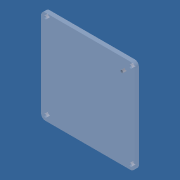
# Autodesk Inventor part: J007954
Saved by Autodesk Inventor 2018.2 (Build 222227000, 227)
## iProperties
Created: 2018-01-11
Material: ACRYLIC, CLEAR
Vendor: HHMI: JRC - ID&F
Document SubType Name: Modeling
Designer: negrashovi
Density: 0.66 g/cm^3
Appearance: Polycarbonate (Clear)
Project: P-159707
Description: WINDOW
Part Number: J007954
RuleStatus: InUse
AfterDocSave0: file://Part Number Cleaner
LAB/DEPT: RUBIN (LAB)
REQUESTING SCIENTIST: ASO, YOSHI
SURFACE ROUGHNESS: N/A
DESIGN DEPARTMENT: HHMI: JRC - ID&F
SPECIAL FINISH: NONE
ALTERED ITEM PART NUMBER: N/A
ALTERED ITEM VENDOR: N/A
ALTERED ITEM DESCRIPTION: N/A
Author: negrashovi
Revision Number: -
Autodesk Inventor part; units mm, degrees
ref_plane "YZ Plane" through (0, 0, 0) normal (1, 0, 0) x (0, 1, 0)
ref_plane "XZ Plane" through (0, 0, 0) normal (0, 1, 0) x (-1, 0, 0)
ref_plane "XY Plane" through (0, 0, 0) normal (0, 0, 1) x (1, 0, 0)
sketch "Sketch1" plane through (0, 0, 0) normal (0, 0, 1) x (1, 0, 0)
  line L0 (-63.5, -69.85) -> (63.5, -69.85)
  line L1 (69.85, -63.5) -> (69.85, 63.5)
  line L2 (63.5, 69.85) -> (-63.5, 69.85)
  line L3 (-69.85, 63.5) -> (-69.85, -63.5)
  arc A0 (-63.5, 69.85) -> (-69.85, 63.5) centre (-63.5, 63.5) ccw
  arc A1 (69.85, 63.5) -> (63.5, 69.85) centre (63.5, 63.5) ccw
  arc A2 (63.5, -69.85) -> (69.85, -63.5) centre (63.5, -63.5) ccw
  arc A3 (-69.85, -63.5) -> (-63.5, -69.85) centre (-63.5, -63.5) ccw
  point P0 (0, 0)
  point P1 (69.85, 0)
  point P2 (0, 69.85)
  point P3 (50.8, 50.8)
  dimension "d0" = 139.7
  dimension "d1" = 139.7
  dimension "d2" = 6.35
  dimension "d3" = 19.05
  dimension "d4" = 19.05
  constraints: 8 end point, 8 point on circle, 8 tangent, 4 centre point, 4 coincident, 3 equal radius, 2 midpoint, 2 parallel, 1 horizontal, 1 horizontal alignment, 1 perpendicular, 1 vertical alignment
  measures "d0" distance between parallel lines of L1 L3
  measures "d1" distance between parallel lines of L0 L2
  measures "d2" radius of A0
  measures "d3" distance from line of point (50.8, 50.8) L1
  measures "d4" distance from line of point (50.8, 50.8) L2
extrude "Extrusion1" add sketch "Sketch1" against normal blind 6.35
hole "Hole1" at (-63.5, 63.5, 0) at (63.5, 63.5, 0) at (63.5, -63.5, 0) at (-63.5, -63.5, 0) direction (0, 0, -1) diameter 4.4958 end through all clearance for "Flat Head Machine Screw (82)" size "#8" standard "Ansi Unified Screw Threads"
hole "Hole2" at (50.8, 50.8, 0) direction (0, 0, -1) diameter 3.9624 end through all thread size "10-32 UNF" class "2B" standard "ANSI Unified Screw Threads"
equation "\"d1\" = d0"
equation "\"d4\" = d3"
body "Solid1"
